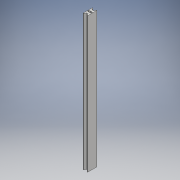
# Autodesk Inventor part: wheelRoadGantry
Saved by Autodesk Inventor 2017 (Build 210142000, 142)
## iProperties
Created: 2016-11-26
Part Number: wheelRoadGantry
Material: Generic
Document SubType Name: Modeling
Designer: umr
Density: 1 g/cm^3
Appearance: Default
Author: umr
Autodesk Inventor part; units mm, degrees
ref_plane "YZ Plane" through (0, 0, 0) normal (1, 0, 0) x (0, 1, 0)
ref_plane "XZ Plane" through (0, 0, 0) normal (0, 1, 0) x (-1, 0, 0)
ref_plane "XY Plane" through (0, 0, 0) normal (0, 0, 1) x (1, 0, 0)
sketch "Sketch1" plane through (0, 0, 0) normal (0, 0, 1) x (1, 0, 0)
  line L0 (0, 0) -> (50, 0)
  line L1 (50, 0) -> (50, 100)
  line L2 (50, 100) -> (0, 100)
  line L3 (0, 100) -> (0, 0)
  dimension "d0" = 50
  dimension "d1" = 100
  constraints: 8 end point, 2 parallel, 1 horizontal, 1 perpendicular
  measures "d0" distance of L2.end L1.end
  measures "d1" distance of L0.end L1.end
extrude "Extrusion1" add sketch "Sketch1" along normal blind 1500
sketch "Sketch2" plane through (0, 0, 1500) normal (0, 0, 1) x (1, 0, 0)
  line L0 (0, 0) -> (50, 0) projected
  line L1 (50, 0) -> (50, 100) projected
  line L2 (50, 100) -> (0, 100) projected
  line L3 (0, 100) -> (0, 0) projected
  line L4 (16.6667, 80) -> (33.3333, 80)
  line L5 (16.6667, 80) -> (43.3333, 80) construction
  line L6 (16.6667, 80) -> (5.1197, 100)
  line L7 (50, 100) -> (0, 100) projected
  line L8 (16.6667, 80) -> (39.7607, 80) construction
  line L9 (33.3333, 80) -> (44.8803, 100)
  line L10 (33.3333, 80) -> (56.4273, 80) construction
  line L11 (44.8803, 100) -> (5.1197, 100)
  line L12 (0, 50) -> (50, 50)
  line L13 (50, 0) -> (50, 100) projected
  line L14 (16.6667, 20) -> (33.3333, 20)
  line L15 (16.6667, 20) -> (5.1197, 0)
  line L16 (33.3333, 20) -> (44.8803, 0)
  line L17 (44.8803, 0) -> (5.1197, 0)
  dimension "d4" = 50
  dimension "d5" = 16.6667
  dimension "d6" = 100
  dimension "d7" = 20
  dimension "d8" = 16.6667
  dimension "d11" = 120
  dimension "d12" = 60
  dimension "d13" = 50
  constraints: 24 end point, 4 horizontal, 4 symmetric about line, 2 equal length, 2 midpoint, 2 point on line, 1 collinear, 1 perpendicular
  measures "d4" distance of L1.end L2.end
  measures "d5" distance of L4.start L4.end
  measures "d6" distance of L0.end L1.end
  measures "d7" distance between parallel lines of L4 L2
  measures "d8" distance from line of L1 L4.end
  measures "d11" angle of L8 L6
  measures "d12" angle of L10 L9
  measures "d13" distance between parallel lines of L0 L12
extrude "Extrusion2" cut sketch "Sketch2" against normal up to next contours L15 L14 L16 L0 | L2 L9 L4 L6
sketch "Sketch3" plane through (0, 0, 1500) normal (0, 0, 1) x (1, 0, 0)
  line L0 (33.3333, 80) -> (16.6667, 80) projected
  line L1 (16.6667, 60) -> (33.3333, 60)
  line L2 (0, 100) -> (0, 0) projected
  line L3 (16.6667, 20) -> (33.3333, 20) projected
  line L4 (50, 100) -> (44.8803, 100) projected
  line L5 (16.6667, 40) -> (33.3333, 40)
  line L6 (5.1197, 56.6667) -> (5.1197, 43.3333)
  line L7 (25, 80) -> (25, 20)
  line L8 (16.6667, 60) -> (5.1197, 56.6667)
  line L9 (16.6667, 40) -> (5.1197, 43.3333)
  line L10 (44.8803, 56.6667) -> (44.8803, 43.3333)
  line L11 (33.3333, 60) -> (44.8803, 56.6667)
  line L12 (33.3333, 40) -> (44.8803, 43.3333)
  dimension "d16" = 16.6667
  dimension "d17" = 16.6667
  dimension "d18" = 16.6667
  dimension "d19" = 16.6667
  dimension "d20" = 20
  dimension "d21" = 20
  dimension "d22" = 100
  dimension "d23" = 16.6667
  dimension "d25" = 40
  dimension "d26" = 16.6667
  dimension "d27" = 13.3333
  dimension "d28" = 3.3333
  constraints: 18 end point, 2 horizontal, 2 midpoint, 2 symmetric about line, 2 vertical
  measures "d16" distance of L0.start L0.end
  measures "d17" distance of L1.start L1.end
  measures "d18" distance from line of L2 L0.end
  measures "d19" distance from line of L2 L1.start
  measures "d20" distance between parallel lines of L4 L0
  measures "d21" distance between parallel lines of L1 L0
  measures "d22" distance of L2.start L2.end
  measures "d23" distance of L5.start L5.end
  measures "d25" distance between parallel lines of L0 L5
  measures "d26" distance from line of L2 L5.start
  measures "d27" distance of L6.start L6.end
  measures "d28" vertical distance of L6.start L1.start
extrude "Extrusion3" cut sketch "Sketch3" against normal blind 2900
equation "\"d1\" = 2 * d0"
equation "\"d5\" = 0.333333 * d4"
equation "\"d7\" = 0.2 * d6"
equation "\"d8\" = -0.5 * d5 + 0.5 * d4"
equation "\"d13\" = 0.5 * d6"
equation "\"d17\" = d16"
equation "\"d19\" = d18"
equation "\"d21\" = 0.5 * d22 - 1.5 * d20"
equation "\"d23\" = d24"
equation "\"d25\" = -0.5 * d20 + 0.5 * d22"
equation "\"d26\" = d16"
equation "\"d27\" = 0.666667 * d21"
equation "\"d28\" = -0.5 * d27 + 0.5 * d21"
equation "\"d24\" = 16.666667"
body "Solid1"
